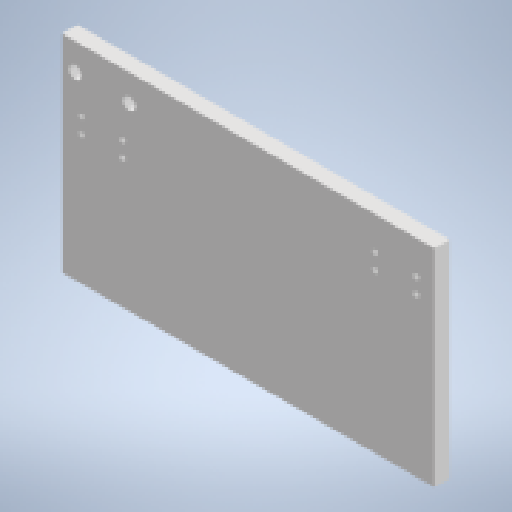
# Autodesk Inventor part: Base de mdf
Saved by Autodesk Inventor 2023 (Build 270158000, 158)
## iProperties
Created: 2022-09-27
Part Number: Base de mdf
Material: Generic
Document SubType Name: Modeling
Designer: kleber
Density: 1 g/cm^3
Appearance: Default
Description: Base de MDF 360x200
Author: kleber
Autodesk Inventor part; units mm, degrees
ref_plane "YZ Plane" through (0, 0, 0) normal (1, 0, 0) x (0, 1, 0)
ref_plane "XZ Plane" through (0, 0, 0) normal (0, 1, 0) x (-1, 0, 0)
ref_plane "XY Plane" through (0, 0, 0) normal (0, 0, 1) x (1, 0, 0)
sketch "Sketch1" plane through (0, 0, 0) normal (0, 0, 1) x (1, 0, 0)
  line L0 (0.6703, -50.425) -> (0.6703, 149.575)
  line L1 (0.6703, 149.575) -> (-359.3297, 149.575)
  line L2 (-359.3297, 149.575) -> (-359.3297, -50.425)
  line L3 (-359.3297, -50.425) -> (0.6703, -50.425)
  line L4 (0.6703, -50.425) -> (0.6703, 149.575)
  point P0 (0, 0)
  dimension "d67" = 360
  constraints: 10 end point, 2 parallel, 1 horizontal, 1 perpendicular
  measures "d67" distance of L3.end L2.end
extrude "Extrusion1" add sketch "Sketch1" along normal blind 15
sketch "Sketch7" plane through (0, 0, 0) normal (0, 0, -1) x (-1, 0, 0)
  line L0 (-0.6703, 149.575) -> (359.3297, 149.575) projected
  line L1 (-0.6703, 149.575) -> (359.3297, 149.575) projected
  line L2 (359.3297, 149.575) -> (359.3297, -50.425) projected
  line L3 (-0.6703, -50.425) -> (-0.6703, 149.575) projected
  line L4 (-0.6703, 149.575) -> (-0.6703, 129.575)
  line L5 (-0.6703, 149.575) -> (-0.6703, 119.575)
  line L6 (-0.6703, 119.575) -> (-0.6703, 117.575)
  circle A0 centre (56.8297, 102.575) radius 1.5
  circle A1 centre (56.8297, 117.575) radius 1.5
  circle A2 centre (21.8297, 102.575) radius 1.5
  circle A3 centre (21.8297, 117.575) radius 1.5
  line L7 (359.3297, 149.575) -> (359.3297, -50.425) projected
  line L8 (-0.6703, 117.575) -> (-0.6703, 119.575)
  line L9 (-0.6703, 117.575) -> (-0.6703, 120.575)
  circle A4 centre (300.6557, 89.6777) radius 1.59
  circle A5 centre (300.6557, 74.6777) radius 1.59
  line L10 (16.8297, 102.575) -> (21.8297, 102.575)
  point P0 (0, 0)
  point P1 (300.6557, 74.6777)
  point P2 (340.6556, 74.6777)
  point P3 (340.6556, 89.6777)
  point P4 (335.6556, 88.0877)
  dimension "d70" = 20
  dimension "d155" = 3
  constraints: 12 end point, 6 centre point, 4 point on line, 1 collinear, 1 horizontal, 4 other
  measures "d70" distance of L0.start L4.end
  measures "d155" distance of L6.end L9.end
hole "Hole10" at (-56.8297, 102.575, 0) at (-56.8297, 117.575, 0) at (-21.8297, 117.575, 0) at (-21.8297, 102.575, 0) direction (0, 0, 1) diameter 3 end through all
hole "Hole11" at (-300.6557, 74.6777, 0) at (-300.6557, 89.6777, 0) at (-340.6556, 74.6777, 0) at (-340.6556, 89.6777, 0) direction (0, 0, 1) diameter 3 end through all
sketch "Sketch11" plane through (0, 0, 15) normal (0, 0, 1) x (1, 0, 0)
  circle A0 centre (-21.8297, 117.575) radius 1.5 projected
  circle A1 centre (-56.8297, 102.575) radius 1.5 projected
  circle A2 centre (-56.8297, 117.575) radius 1.5 projected
  circle A3 centre (-21.8297, 102.575) radius 1.5 projected
  line L0 (0.6703, -50.425) -> (0.6703, 149.575) projected
  line L1 (0.6703, 149.575) -> (-359.3297, 149.575) projected
  line L2 (-359.3297, 149.575) -> (-359.3297, -50.425) projected
  line L3 (-359.3297, -50.425) -> (0.6703, -50.425) projected
  circle A4 centre (-56.8297, 102.575) radius 1.5 projected
  circle A5 centre (-340.6556, 74.6777) radius 1.5 projected
  circle A6 centre (-340.6556, 89.6777) radius 1.5 projected
  circle A7 centre (-340.6556, 74.6777) radius 1.5 projected
  circle A8 centre (-300.6557, 74.6777) radius 1.5 projected
  circle A9 centre (-300.6557, 89.6777) radius 1.5 projected
  circle A10 centre (-340.6556, 89.6777) radius 1.5 projected
  circle A11 centre (-21.8297, 117.575) radius 1.5 projected
  circle A12 centre (-56.8297, 102.575) radius 1.5 projected
  circle A13 centre (-56.8297, 117.575) radius 1.5 projected
  circle A14 centre (-21.8297, 102.575) radius 1.5 projected
  line L4 (0.6703, -50.425) -> (0.6703, 149.575) projected
  line L5 (0.6703, 149.575) -> (-359.3297, 149.575) projected
  line L6 (-359.3297, 149.575) -> (-359.3297, -50.425) projected
  line L7 (-359.3297, -50.425) -> (0.6703, -50.425) projected
  point P0 (0, 0)
hole "Hole12" at (-56.8297, 117.575, 15) at (-56.8297, 102.575, 15) at (-21.8297, 102.575, 15) at (-21.8297, 117.575, 15) at (-300.6557, 74.6777, 15) at (-300.6557, 89.6777, 15) at (-340.6556, 89.6777, 15) at (-340.6556, 74.6777, 15) direction (0, 0, -1) diameter 3 end through all countersink diameter 6 countersink angle 90
sketch "Sketch12" plane through (0, 0, 0) normal (0, 0, -1) x (-1, 0, 0)
  circle A0 centre (294.6557, 123.5777) radius 4
  circle A1 centre (346.6557, 123.5777) radius 4
  point P0 (0, 0)
  constraints: 2 centre point, 4 other
hole "Hole13" at (-294.6557, 123.5777, 0) at (-346.6557, 123.5777, 0) direction (0, 0, 1) diameter 8 end through all
sketch "Sketch13" plane through (0, 0, 15) normal (0, 0, 1) x (1, 0, 0)
  circle A0 centre (-346.6557, 123.5777) radius 4 projected
  circle A1 centre (-294.6557, 123.5777) radius 4 projected
  point P0 (0, 0)
hole "Hole14" at (-346.6557, 123.5777, 15) at (-294.6557, 123.5777, 15) direction (0, 0, -1) diameter 12 depth 8
body "Solid1"
